Autodesk Fusion 360 part; units mm, degrees
note: some values were not read from the file. Set by a fixed rule: which sketch regions a step uses.
(part 2 of 4)
sketch "Sketch8" plane through (0, 57, 0) normal (0, 1, 0) x (0, 0, 1)
  circle A0 centre (-6, 81) radius 8
  circle A1 centre (-6, 61) radius 8
  circle A2 centre (0, 35) radius 14
  circle A3 centre (0, 0) radius 14
  line L0 (-3, 62.5) -> (-9, 62.5)
  line L1 (-9, 62.5) -> (-9, 59.5)
  line L2 (-9, 59.5) -> (-3, 59.5)
  line L3 (-3, 59.5) -> (-3, 62.5)
  line L4 (-3, 82.5) -> (-9, 82.5)
  line L5 (-3, 79.5) -> (-3, 82.5)
  line L6 (-9, 79.5) -> (-3, 79.5)
  line L7 (-9, 82.5) -> (-9, 79.5)
  arc A4 (3.3646, 47.557) -> (-3.3646, 47.557) centre (0, 35) ccw
  line L8 (-1.1647, 39.3467) -> (-3.3646, 47.557)
  line L9 (1.1647, 39.3467) -> (3.3646, 47.557)
  arc A5 (1.1647, 39.3467) -> (-1.1647, 39.3467) centre (0, 35) ccw
  arc A6 (3.8971, 37.25) -> (2.25, 38.8971) centre (0, 35) ccw
  line L10 (2.25, 38.8971) -> (6.5, 46.2583)
  arc A7 (11.2583, 41.5) -> (6.5, 46.2583) centre (0, 35) ccw
  line L11 (3.8971, 37.25) -> (11.2583, 41.5)
  line L12 (4.3467, 36.1647) -> (12.557, 38.3646)
  arc A8 (12.557, 31.6354) -> (12.557, 38.3646) centre (0, 35) ccw
  line L13 (4.3467, 33.8353) -> (12.557, 31.6354)
  arc A9 (4.3467, 33.8353) -> (4.3467, 36.1647) centre (0, 35) ccw
  arc A10 (-11.2583, 28.5) -> (-6.5, 23.7417) centre (0, 35) ccw
  arc A11 (-3.3646, 22.443) -> (3.3646, 22.443) centre (0, 35) ccw
  arc A12 (6.5, 23.7417) -> (11.2583, 28.5) centre (0, 35) ccw
  line L14 (3.8971, 32.75) -> (11.2583, 28.5)
  arc A13 (2.25, 31.1029) -> (3.8971, 32.75) centre (0, 35) ccw
  line L15 (2.25, 31.1029) -> (6.5, 23.7417)
  arc A14 (-1.1647, 30.6533) -> (1.1647, 30.6533) centre (0, 35) ccw
  line L16 (1.1647, 30.6533) -> (3.3646, 22.443)
  line L17 (-1.1647, 30.6533) -> (-3.3646, 22.443)
  line L18 (-2.25, 31.1029) -> (-6.5, 23.7417)
  line L19 (-3.8971, 32.75) -> (-11.2583, 28.5)
  arc A15 (-3.8971, 32.75) -> (-2.25, 31.1029) centre (0, 35) ccw
  arc A16 (-4.3467, 36.1647) -> (-4.3467, 33.8353) centre (0, 35) ccw
  line L20 (-4.3467, 33.8353) -> (-12.557, 31.6354)
  line L21 (-4.3467, 36.1647) -> (-12.557, 38.3646)
  arc A17 (-12.557, 38.3646) -> (-12.557, 31.6354) centre (0, 35) ccw
  arc A18 (-6.5, 46.2583) -> (-11.2583, 41.5) centre (0, 35) ccw
  line L22 (-2.25, 38.8971) -> (-6.5, 46.2583)
  line L23 (-3.8971, 37.25) -> (-11.2583, 41.5)
  arc A19 (-2.25, 38.8971) -> (-3.8971, 37.25) centre (0, 35) ccw
  line L24 (3, 36.5) -> (-3, 36.5)
  line L25 (-3, 36.5) -> (-3, 33.5)
  line L26 (-3, 33.5) -> (3, 33.5)
  line L27 (3, 33.5) -> (3, 36.5)
  arc A20 (-3.8971, -2.25) -> (-2.25, -3.8971) centre (0, 0) ccw
  arc A21 (-1.1647, -4.3467) -> (1.1647, -4.3467) centre (0, 0) ccw
  arc A22 (2.25, -3.8971) -> (3.8971, -2.25) centre (0, 0) ccw
  arc A23 (4.3467, -1.1647) -> (4.3467, 1.1647) centre (0, 0) ccw
  arc A24 (3.8971, 2.25) -> (2.25, 3.8971) centre (0, 0) ccw
  arc A25 (1.1647, 4.3467) -> (-1.1647, 4.3467) centre (0, 0) ccw
  arc A26 (-2.25, 3.8971) -> (-3.8971, 2.25) centre (0, 0) ccw
  arc A27 (-4.3467, 1.1647) -> (-4.3467, -1.1647) centre (0, 0) ccw
  line L28 (-4.3467, -1.1647) -> (-12.557, -3.3646)
  line L29 (-4.3467, 1.1647) -> (-12.557, 3.3646)
  arc A28 (-12.557, 3.3646) -> (-12.557, -3.3646) centre (0, 0) ccw
  line L30 (-3.8971, -2.25) -> (-11.2583, -6.5)
  arc A29 (-11.2583, -6.5) -> (-6.5, -11.2583) centre (0, 0) ccw
  line L31 (-2.25, -3.8971) -> (-6.5, -11.2583)
  line L32 (-1.1647, -4.3467) -> (-3.3646, -12.557)
  arc A30 (-3.3646, -12.557) -> (3.3646, -12.557) centre (0, 0) ccw
  line L33 (1.1647, -4.3467) -> (3.3646, -12.557)
  line L34 (2.25, -3.8971) -> (6.5, -11.2583)
  arc A31 (6.5, -11.2583) -> (11.2583, -6.5) centre (0, 0) ccw
  line L35 (3.8971, -2.25) -> (11.2583, -6.5)
  line L36 (4.3467, -1.1647) -> (12.557, -3.3646)
  line L37 (4.3467, 1.1647) -> (12.557, 3.3646)
  arc A32 (12.557, -3.3646) -> (12.557, 3.3646) centre (0, 0) ccw
  line L38 (3.8971, 2.25) -> (11.2583, 6.5)
  line L39 (2.25, 3.8971) -> (6.5, 11.2583)
  line L40 (1.1647, 4.3467) -> (3.3646, 12.557)
  line L41 (-1.1647, 4.3467) -> (-3.3646, 12.557)
  line L42 (-2.25, 3.8971) -> (-6.5, 11.2583)
  line L43 (-3.8971, 2.25) -> (-11.2583, 6.5)
  arc A33 (-6.5, 11.2583) -> (-11.2583, 6.5) centre (0, 0) ccw
  arc A34 (3.3646, 12.557) -> (-3.3646, 12.557) centre (0, 0) ccw
  arc A35 (11.2583, 6.5) -> (6.5, 11.2583) centre (0, 0) ccw
  circle A36 centre (0, -35) radius 14
  line L44 (3, -33.5) -> (-3, -33.5)
  line L45 (-3, -33.5) -> (-3, -36.5)
  line L46 (-3, -36.5) -> (3, -36.5)
  line L47 (3, -36.5) -> (3, -33.5)
  arc A37 (4.3467, -36.1647) -> (4.3467, -33.8353) centre (0, -35) ccw
  line L48 (4.3467, -33.8353) -> (12.557, -31.6354)
  arc A38 (12.557, -38.3646) -> (12.557, -31.6354) centre (0, -35) ccw
  line L49 (4.3467, -36.1647) -> (12.557, -38.3646)
  line L50 (3.8971, -37.25) -> (11.2583, -41.5)
  arc A39 (2.25, -38.8971) -> (3.8971, -37.25) centre (0, -35) ccw
  line L51 (2.25, -38.8971) -> (6.5, -46.2583)
  arc A40 (6.5, -46.2583) -> (11.2583, -41.5) centre (0, -35) ccw
  arc A41 (-3.3646, -47.557) -> (3.3646, -47.557) centre (0, -35) ccw
  line L52 (-1.1647, -39.3467) -> (-3.3646, -47.557)
  arc A42 (-1.1647, -39.3467) -> (1.1647, -39.3467) centre (0, -35) ccw
  line L53 (1.1647, -39.3467) -> (3.3646, -47.557)
  line L54 (-2.25, -38.8971) -> (-6.5, -46.2583)
  arc A43 (-11.2583, -41.5) -> (-6.5, -46.2583) centre (0, -35) ccw
  line L55 (-3.8971, -37.25) -> (-11.2583, -41.5)
  arc A44 (-3.8971, -37.25) -> (-2.25, -38.8971) centre (0, -35) ccw
  line L56 (-4.3467, -36.1647) -> (-12.557, -38.3646)
  arc A45 (-12.557, -31.6354) -> (-12.557, -38.3646) centre (0, -35) ccw
  line L57 (-4.3467, -33.8353) -> (-12.557, -31.6354)
  arc A46 (-4.3467, -33.8353) -> (-4.3467, -36.1647) centre (0, -35) ccw
  arc A47 (-2.25, -31.1029) -> (-3.8971, -32.75) centre (0, -35) ccw
  arc A48 (1.1647, -30.6533) -> (-1.1647, -30.6533) centre (0, -35) ccw
  arc A49 (3.8971, -32.75) -> (2.25, -31.1029) centre (0, -35) ccw
  line L58 (-3.8971, -32.75) -> (-11.2583, -28.5)
  arc A50 (-6.5, -23.7417) -> (-11.2583, -28.5) centre (0, -35) ccw
  line L59 (-2.25, -31.1029) -> (-6.5, -23.7417)
  line L60 (-1.1647, -30.6533) -> (-3.3646, -22.443)
  arc A51 (3.3646, -22.443) -> (-3.3646, -22.443) centre (0, -35) ccw
  line L61 (1.1647, -30.6533) -> (3.3646, -22.443)
  line L62 (2.25, -31.1029) -> (6.5, -23.7417)
  arc A52 (11.2583, -28.5) -> (6.5, -23.7417) centre (0, -35) ccw
  line L63 (3.8971, -32.75) -> (11.2583, -28.5)
  circle A53 centre (-6, -81) radius 8
  circle A54 centre (-6, -61) radius 8
  line L64 (-9, -59.5) -> (-9, -62.5)
  line L65 (-3, -59.5) -> (-9, -59.5)
  line L66 (-3, -62.5) -> (-3, -59.5)
  line L67 (-9, -62.5) -> (-3, -62.5)
  line L68 (-3, -79.5) -> (-9, -79.5)
  line L69 (-3, -82.5) -> (-3, -79.5)
  line L70 (-9, -82.5) -> (-3, -82.5)
  line L71 (-9, -79.5) -> (-9, -82.5)
  line L72 (3, 1.5) -> (3, -1.5)
  line L73 (3, -1.5) -> (-3, -1.5)
  line L74 (-3, -1.5) -> (-3, 1.5)
  line L75 (-3, 1.5) -> (3, 1.5)
extrude "Extrude28" add sketch "Sketch8" along normal blind 3 separate body contours A0 makes body 28
extrude "Extrude29" add sketch "Sketch8" along normal blind 3 separate body contours A1 makes body 29
extrude "Extrude30" add sketch "Sketch8" along normal blind 3 separate body contours A2 makes body 30
extrude "Extrude31" add sketch "Sketch8" along normal blind 3 separate body contours A3 makes body 31
extrude "Extrude32" add sketch "Sketch8" along normal blind 3 separate body contours A36 makes body 32
extrude "Extrude33" add sketch "Sketch8" along normal blind 3 separate body contours A54 makes body 33
extrude "Extrude34" add sketch "Sketch8" along normal blind 3 separate body contours A53 makes body 34
ref_plane "WorkPlane8" through (-61, 60, -6) normal (0, 1, 0) x (0, 0, 1)
sketch "Sketch9" plane through (0, 60, 0) normal (0, 1, 0) x (0, 0, 1)
  line L0 (-6, 82.5) -> (-6, 84.5)
  arc A0 (-5, 85.5) -> (-6, 84.5) centre (-5, 84.5) ccw
  line L1 (0, 85.5) -> (-5, 85.5)
  arc A1 (3, 82.5) -> (0, 85.5) centre (0, 82.5) ccw
  line L2 (3, 59.5) -> (3, 82.5)
  arc A2 (0, 56.5) -> (3, 59.5) centre (0, 59.5) ccw
  line L3 (-5, 56.5) -> (0, 56.5)
  line L4 (-6, 59.5) -> (-6, 57.5)
  arc A3 (-6, 57.5) -> (-5, 56.5) centre (-5, 57.5) ccw
  line L5 (-6, 62.5) -> (-6, 79.5)
  line L6 (-3, 79.5) -> (-3, 82.5)
  line L7 (-3, 59.5) -> (-3, 62.5)
  line L8 (-6, -59.5) -> (-6, -57.5)
  arc A4 (-5, -56.5) -> (-6, -57.5) centre (-5, -57.5) ccw
  line L9 (0, -56.5) -> (-5, -56.5)
  line L10 (-3, -62.5) -> (-3, -59.5)
  arc A5 (3, -59.5) -> (0, -56.5) centre (0, -59.5) ccw
  line L11 (3, -82.5) -> (3, -59.5)
  line L12 (-6, -79.5) -> (-6, -62.5)
  line L13 (-3, -82.5) -> (-3, -79.5)
  line L14 (-6, -82.5) -> (-6, -84.5)
  arc A6 (-6, -84.5) -> (-5, -85.5) centre (-5, -84.5) ccw
  line L15 (-5, -85.5) -> (0, -85.5)
  arc A7 (0, -85.5) -> (3, -82.5) centre (0, -82.5) ccw
  line L16 (-3, 82.5) -> (-6, 82.5)
  line L17 (-3, 79.5) -> (-6, 79.5)
  line L18 (-3, 62.5) -> (-6, 62.5)
  line L19 (-3, 59.5) -> (-6, 59.5)
  line L20 (-3, -59.5) -> (-6, -59.5)
  line L21 (-3, -62.5) -> (-6, -62.5)
  line L22 (-3, -79.5) -> (-6, -79.5)
  line L23 (-3, -82.5) -> (-6, -82.5)
  arc A8 (14.7459, 42.5217) -> (16.2941, 44.7585) centre (15, 44) ccw
  line L24 (3.3176, 38.2212) -> (14.7459, 42.5217)
  line L25 (2.2907, 39.2175) -> (15, 44)
  arc A9 (2.2907, 39.2175) -> (-0.2332, 37.8932) centre (1.2462, 38.1409) ccw
  line L26 (0, 36.5) -> (-0.2332, 37.8932)
  line L27 (2.9851, 36.5) -> (0, 36.5)
  line L28 (2.9851, 36.5) -> (2.9851, 33.5)
  line L29 (2.9851, 33.5) -> (0.5022, 33.5)
  arc A10 (0.5208, 33.389) -> (1.0114, 32.179) centre (3.4796, 33.8843) ccw
  line L30 (0.5208, 33.389) -> (0.5022, 33.5)
  line L31 (5.5685, 36.0375) -> (3.3176, 38.2212)
  arc A11 (2.3055, 31.1236) -> (5.5685, 36.0375) centre (3.4796, 33.8843) ccw
  line L32 (2.3055, 4.2031) -> (2.3055, 31.1236)
  line L33 (1.0114, 4.6224) -> (1.0114, 32.179)
  line L34 (2.9851, 1.5) -> (0, 1.5)
  line L35 (0, 1.5) -> (-0.2332, 2.8932)
  arc A12 (1.0114, 4.6224) -> (-0.2332, 2.8932) centre (1.2462, 3.1409) ccw
  line L36 (5.5685, 1.0375) -> (2.2907, 4.2175)
  arc A13 (2.3055, -3.8764) -> (5.5685, 1.0375) centre (3.4796, -1.1157) ccw
  line L37 (2.9851, 1.5) -> (2.9851, -1.5)
  line L38 (2.9851, -1.5) -> (0.5022, -1.5)
  arc A14 (0.5208, -1.611) -> (1.0114, -2.821) centre (3.4796, -1.1157) ccw
  line L39 (0.5208, -1.611) -> (0.5022, -1.5)
  line L40 (1.0114, -30.38) -> (1.0114, -2.821)
  line L41 (2.3055, -30.7825) -> (2.3055, -3.8764)
  line L42 (0.0149, -33.5) -> (-0.2184, -32.1068)
  arc A15 (1.0114, -30.38) -> (-0.2184, -32.1068) centre (1.261, -31.8591) ccw
  line L43 (5.5834, -33.9625) -> (2.3055, -30.7825)
  line L44 (3, -33.5) -> (0.0149, -33.5)
  line L45 (3, -33.5) -> (3, -36.5)
  line L46 (3, -36.5) -> (0.517, -36.5)
  arc A16 (0.5356, -36.611) -> (5.5834, -33.9625) centre (3.4944, -36.1157) ccw
  line L47 (0.5356, -36.611) -> (0.517, -36.5)
  line L48 (15, 78) -> (16.2941, 78)
  line L49 (16.2941, 78) -> (16.2941, 44.7585)
  line L50 (15, 78) -> (15, 44)
  constraint coincident L6.end L16.start
  constraint coincident L0.start L16.end
  constraint coincident L6.start L17.start
  constraint coincident L5.end L17.end
  constraint coincident L7.end L18.start
  constraint coincident L5.start L18.end
  constraint coincident L7.start L19.start
  constraint coincident L4.start L19.end
  constraint coincident L10.end L20.start
  constraint coincident L8.start L20.end
  constraint coincident L10.start L21.start
  constraint coincident L12.end L21.end
  constraint coincident L13.end L22.start
  constraint coincident L12.start L22.end
  constraint coincident L13.start L23.start
  constraint coincident L14.start L23.end
  constraint coincident A8.end L49.end
  constraint perpendicular L48 L49
  constraint coincident A8.centre L25.end
  constraint perpendicular L48 L50
extrude "Extrude35" add sketch "Sketch9" along normal blind 3 separate body contours L8 A4 L9 L10 A5 L11 L12 L13 L14 A6 L15 A7 L20 L21 L22 L23 makes body 35
extrude "Extrude36" add sketch "Sketch9" along normal blind 3 separate body contours L0 A0 L1 A1 L2 A2 L3 L4 A3 L5 L6 L7 L16 L17 L18 L19 makes body 36
extrude "Extrude37" add sketch "Sketch9" along normal blind 3 separate body contours A8 L24 L25 A9 L26 L27 L28 L29 A10 L30 L31 A11 L32 L33 L34 L35 A12 L36 A13 L37 L38 A14 L39 L40 L41 L42 A15 L43 L44 L45 L46 A16 L47 L48 L49 L50 makes body 37
ref_plane "WorkPlane9" through (-59.5, -6, 11.5) normal (0, -1, 0) x (1, 0, 0)
sketch "Sketch10" plane through (0, -6, 0) normal (0, -1, 0) x (1, 0, 0)
  line L0 (-61, 10) -> (-61, 13)
  line L1 (-58, 10) -> (-61, 10)
  line L2 (-58, 10) -> (-58, 13)
  line L3 (-58, 13) -> (-55, 13)
  line L4 (-93, 10) -> (-93, 13)
  line L5 (-93, 10) -> (-90, 10)
  line L6 (-90, 10) -> (-90, 13)
  line L7 (-98, 13) -> (-93, 13)
  line L8 (-90, 13) -> (-61, 13)
  line L9 (-55, 13) -> (-55, 18)
  line L10 (-55, 68) -> (-58, 68)
  line L11 (-58, 68) -> (-58, 65)
  line L12 (-58, 65) -> (-55, 65)
  line L13 (-55, 18) -> (-58, 18)
  line L14 (-58, 18) -> (-58, 21)
  line L15 (-58, 21) -> (-55, 21)
  line L16 (-55, 65) -> (-55, 21)
  line L17 (-98, 13) -> (-98, 18)
  line L18 (-98, 18) -> (-95, 18)
  line L19 (-95, 18) -> (-95, 21)
  line L20 (-95, 21) -> (-98, 21)
  line L21 (-98, 65) -> (-98, 21)
  line L22 (-95, 65) -> (-98, 65)
  line L23 (-95, 68) -> (-95, 65)
  line L24 (-98, 68) -> (-95, 68)
  line L25 (-88.5, 67.3205) -> (-64.5, 67.3205)
  arc A0 (-88.5, 67.3205) -> (-91.5, 64.3205) centre (-88.5, 64.3205) ccw
  arc A1 (-61.5, 64.3205) -> (-64.5, 67.3205) centre (-64.5, 64.3205) ccw
  line L26 (-91.5, 64.3205) -> (-91.5, 47.3205)
  line L27 (-61.5, 64.3205) -> (-61.5, 47.3205)
  line L28 (-64.5, 44.3205) -> (-88.5, 44.3205)
  arc A2 (-91.5, 47.3205) -> (-88.5, 44.3205) centre (-88.5, 47.3205) ccw
  arc A3 (-64.5, 44.3205) -> (-61.5, 47.3205) centre (-64.5, 47.3205) ccw
  line L29 (-98, 68) -> (-98, 70)
  line L30 (-55, 68) -> (-55, 70)
  line L31 (-55, 70) -> (-98, 70)
  point P0 (-93, 68)
  point P1 (-60, 68)
  point P2 (-60, 29)
  point P3 (-93, 29)
  point P4 (-91.5, 67.3205)
  point P5 (-61.5, 67.3205)
  point P6 (-91.5, 44.3205)
  point P7 (-61.5, 44.3205)
  dimension "d185" = 39
  dimension "d186" = 39
  dimension "d191" = 5
  dimension "d193" = 3
  dimension "d194" = 3
  dimension "d195" = 3
  dimension "d197" = 3
  dimension "d198" = 3
  dimension "d199" = 30
  dimension "d202" = 3
  dimension "d203" = 3
  dimension "d208" = 20
  dimension "d209" = 20
  dimension "d210" = 3
  dimension "d211" = 3
  dimension "d271" = 2
  dimension "d272" = 2
  constraint coincident L3.end L9.start
  constraint perpendicular L3 L9
  constraint perpendicular L10 L11
  constraint perpendicular L11 L12
  constraint horizontal L13
  constraint perpendicular L13 L14
  constraint perpendicular L14 L15
  constraint horizontal L25
  constraint coincident P4 L25
  constraint tangent L25 A0
  constraint coincident P5 L25
  constraint tangent L25 A1
  constraint vertical L26
  constraint vertical L27
  constraint perpendicular L26 L28
  constraint coincident P6 L26
  constraint coincident P6 L28
  constraint tangent L26 A2
  constraint tangent L28 A2
  constraint coincident P7 L28
  constraint coincident P7 L27
  constraint tangent L28 A3
  constraint tangent L27 A3
  constraint perpendicular L24 L29
  measures "d185" distance of P1 P2
  measures "d186" distance of P0 P3
  measures "d191" distance of L3.end L9.end
  measures "d193" distance of L10.start L10.end
  measures "d194" distance of L10.end L11.end
  measures "d195" distance of L11.end L12.end
  measures "d197" distance of L9.end L13.end
  measures "d198" distance of L14.end L15.end
  measures "d199" distance of P4 P5
  measures "d202" radius of A0
  measures "d203" radius of A1
  measures "d208" distance of A0.end P6
  measures "d209" distance of A1.start P7
  measures "d210" radius of A2
  measures "d211" radius of A3
  measures "d271" distance of L24.start L29.end
  measures "d272" distance of L10.start L30.end
extrude "Extrude38" add sketch "Sketch10" along normal blind 3 separate body makes body 38
ref_plane "WorkPlane10" through (-61.5, 60, 11.5) normal (0, 1, 0) x (-1, 0, 0)
sketch "Sketch11" plane through (0, 60, 0) normal (0, 1, 0) x (-1, 0, 0)
  arc A0 (91.5, 64.3205) -> (88.5, 67.3205) centre (88.5, 64.3205) ccw
  line L0 (91.5, 64.3205) -> (91.5, 47.3205)
  arc A1 (88.5, 44.3205) -> (91.5, 47.3205) centre (88.5, 47.3205) ccw
  line L1 (88.5, 44.3205) -> (64.5, 44.3205)
  arc A2 (61.5, 47.3205) -> (64.5, 44.3205) centre (64.5, 47.3205) ccw
  line L2 (61.5, 47.3205) -> (61.5, 64.3205)
  arc A3 (64.5, 67.3205) -> (61.5, 64.3205) centre (64.5, 64.3205) ccw
  line L3 (64.5, 67.3205) -> (88.5, 67.3205)
  line L4 (55, 68) -> (58, 68)
  line L5 (58, 68) -> (58, 65)
  line L6 (58, 65) -> (55, 65)
  line L7 (55, 65) -> (55, 21)
  line L8 (55, 21) -> (58, 21)
  line L9 (58, 21) -> (58, 18)
  line L10 (58, 18) -> (55, 18)
  line L11 (55, 18) -> (55, 13)
  line L12 (55, 13) -> (58, 13)
  line L13 (58, 13) -> (58, 10)
  line L14 (58, 10) -> (61, 10)
  line L15 (61, 10) -> (61, 13)
  line L16 (61, 13) -> (90, 13)
  line L17 (90, 13) -> (90, 10)
  line L18 (90, 10) -> (93, 10)
  line L19 (93, 10) -> (93, 13)
  line L20 (93, 13) -> (98, 13)
  line L21 (98, 13) -> (98, 18)
  line L22 (98, 18) -> (95, 18)
  line L23 (95, 18) -> (95, 21)
  line L24 (95, 21) -> (98, 21)
  line L25 (98, 21) -> (98, 65)
  line L26 (98, 65) -> (95, 65)
  line L27 (95, 65) -> (95, 68)
  line L28 (95, 68) -> (98, 68)
  line L29 (55, 68) -> (55, 70)
  line L30 (98, 68) -> (98, 70)
  line L31 (98, 70) -> (55, 70)
  line L32 (55, 70) -> (55, 68)
  line L33 (98, 68) -> (98, 70)
  line L34 (98, 70) -> (55, 70)
  dimension "d269" = 2
  dimension "d270" = 2
  constraint coincident L4.start L29.start
  constraint perpendicular L6 L29
  constraint coincident L28.end L30.start
  constraint perpendicular L28 L30
  measures "d269" distance of L4.start L29.end
  measures "d270" distance of L28.end L30.end
extrude "Extrude39" add sketch "Sketch11" along normal blind 3 separate body makes body 39
ref_plane "WorkPlane11" through (-95, -7.5, 66.5) normal (-1, 0, 0) x (0, 0, -1)
sketch "Sketch12" plane through (-95, 0, 0) normal (-1, 0, 0) x (0, 0, -1)
  line L0 (-18, -63) -> (-21, -63)
  line L1 (-21, -60) -> (-21, -63)
  line L2 (-18, -60) -> (-18, -63)
  line L3 (-13, -60) -> (-18, -60)
  line L4 (-10, -58) -> (-13, -58)
  line L5 (-10, -58) -> (-10, -55)
  line L6 (-10, -55) -> (-13, -55)
  line L7 (-13, -55) -> (-13, -28.5)
  line L8 (-13, -25.5) -> (-13, 1)
  line L9 (-10, 1) -> (-13, 1)
  line L10 (-10, 4) -> (-10, 1)
  line L11 (-10, 4) -> (-13, 4)
  line L12 (-13, 6) -> (-18, 6)
  line L13 (-18, 6) -> (-18, 9)
  line L14 (-21, 9) -> (-18, 9)
  line L15 (-21, 6) -> (-21, 9)
  line L16 (-65, 6) -> (-65, 9)
  line L17 (-68, 9) -> (-65, 9)
  line L18 (-68, 6) -> (-68, 9)
  line L19 (-73, 6) -> (-68, 6)
  line L20 (-65, -60) -> (-65, -63)
  line L21 (-65, -63) -> (-68, -63)
  line L22 (-68, -60) -> (-68, -63)
  line L23 (-13, -28.5) -> (-7, -28.5)
  line L24 (-7, -28.5) -> (-7, -25.5)
  line L25 (-13, -25.5) -> (-7, -25.5)
  line L26 (-13, -55) -> (-13, -28.5)
  line L27 (-13, 1) -> (-13, -25.5)
  line L28 (-79.7175, -57.5251) -> (-77.5962, -59.6464)
  line L29 (-77.5962, -59.6464) -> (-75.4749, -57.5251)
  line L30 (-79.7175, -57.5251) -> (-77.5962, -55.4038)
  line L31 (-73, -60) -> (-75.4749, -57.5251)
  line L32 (-77.5962, -55.4038) -> (-80.0711, -52.9289)
  line L33 (-84.1542, -47.0486) -> (-83.6333, -50.003)
  line L34 (-84.1542, -47.0486) -> (-81.1998, -46.5277)
  line L35 (-83.6333, -50.003) -> (-80.6788, -49.4821)
  line L36 (-80.0711, -52.9289) -> (-80.6788, -49.4821)
  line L37 (-81.1998, -46.5277) -> (-81.8075, -43.0809)
  line L38 (-77.5962, 5.6464) -> (-75.4749, 3.5251)
  line L39 (-79.7175, 3.5251) -> (-77.5962, 5.6464)
  line L40 (-79.7175, 3.5251) -> (-77.5962, 1.4038)
  line L41 (-83.6333, -3.9969) -> (-80.6788, -4.5179)
  line L42 (-84.1542, -6.9514) -> (-83.6333, -3.9969)
  line L43 (-84.1542, -6.9514) -> (-81.1998, -7.4723)
  line L44 (-84.8075, -28.5) -> (-84.8075, -25.5)
  line L45 (-84.8075, -25.5) -> (-81.8075, -25.5)
  line L46 (-84.8075, -28.5) -> (-81.8075, -28.5)
  line L47 (-81.8075, -43.0809) -> (-81.8075, -28.5)
  line L48 (-81.8075, -25.5) -> (-81.8075, -10.9191)
  line L49 (-80.0711, -1.0711) -> (-80.6788, -4.5179)
  line L50 (-81.1998, -7.4723) -> (-81.8075, -10.9191)
  line L51 (-73, 6) -> (-75.4749, 3.5251)
  line L52 (-77.5962, 1.4038) -> (-80.0711, -1.0711)
  line L53 (-21, -60) -> (-65, -60)
  line L54 (-65, 6) -> (-21, 6)
  line L55 (-73, 6) -> (-68, 6)
  line L56 (-68, -60) -> (-73, -60)
  line L57 (-13, -60) -> (-13, -58)
  line L58 (-13, 4) -> (-13, 6)
  dimension "d222" = 3
  dimension "d224" = 10
  dimension "d226" = 10
  dimension "d228" = 10
  dimension "d230" = 10
  dimension "d233" = 3
  dimension "d236" = 3
  dimension "d240" = 3
  constraint coincident L7.end L23.start
  constraint perpendicular L7 L23
  constraint perpendicular L23 L24
  constraint coincident L8.start L25.start
  constraint coincident L6.end L7.start
  constraint coincident L8.end L9.end
  constraint coincident L19.start L51.start
  constraint perpendicular L29 L31
  constraint coincident L30.end L31
  constraint perpendicular L30 L31
  constraint collinear L31 L32
  constraint coincident L34.end L36
  constraint perpendicular L34 L36
  constraint perpendicular L35 L36
  constraint collinear L36 L37
  constraint vertical L44
  constraint coincident L45.end L47
  constraint perpendicular L45 L47
  constraint perpendicular L46 L47
  constraint collinear L47 L48
  constraint collinear L49 L50
  constraint collinear L51 L52
  constraint coincident L1.start L53.start
  constraint coincident L20.start L53.end
  constraint coincident L16.start L54.start
  constraint coincident L15.start L54.end
  constraint coincident L18.start L19.end
  constraint coincident L22.start L56.start
  constraint perpendicular L22 L56
  constraint coincident L3.start L57.start
  constraint coincident L4.end L57.end
  constraint coincident L11.end L58.start
  constraint coincident L12.start L58.end
  measures "d222" distance of L23.end L24.end
  measures "d224" distance of L31.start L32.end
  measures "d226" distance of L19.start L49.start
  measures "d228" distance of L32.end L37.end
  measures "d230" distance of L49.start L48.end
  measures "d233" distance of L28.start L28.end
  measures "d236" distance of L33.start L33.end
  measures "d240" distance of L44.start L44.end
extrude "Extrude40" add sketch "Sketch12" along normal blind 3 separate body makes body 40
ref_plane "WorkPlane12" through (-58, -7.5, 66.5) normal (1, 0, 0) x (0, 0, 1)
sketch "Sketch13" plane through (-58, 0, 0) normal (1, 0, 0) x (0, 0, 1)
  line L0 (13, -60) -> (18, -60)
  line L1 (18, -60) -> (18, -63)
  line L2 (18, -63) -> (21, -63)
  line L3 (21, -63) -> (21, -60)
  line L4 (21, -60) -> (65, -60)
  line L5 (65, -60) -> (65, -63)
  line L6 (65, -63) -> (68, -63)
  line L7 (68, -63) -> (68, -60)
  line L8 (68, -60) -> (73, -60)
  line L9 (73, -60) -> (75.4749, -57.5251)
  line L10 (75.4749, -57.5251) -> (77.5962, -59.6464)
  line L11 (77.5962, -59.6464) -> (79.7175, -57.5251)
  line L12 (79.7175, -57.5251) -> (77.5962, -55.4038)
  line L13 (77.5962, -55.4038) -> (80.0711, -52.9289)
  line L14 (80.0711, -52.9289) -> (80.6788, -49.4821)
  line L15 (80.6788, -49.4821) -> (83.6333, -50.003)
  line L16 (83.6333, -50.003) -> (84.1542, -47.0486)
  line L17 (84.1542, -47.0486) -> (81.1998, -46.5277)
  line L18 (81.1998, -46.5277) -> (81.8075, -43.0809)
  line L19 (81.8075, -43.0809) -> (81.8075, -28.5)
  line L20 (81.8075, -28.5) -> (84.8075, -28.5)
  line L21 (84.8075, -28.5) -> (84.8075, -25.5)
  line L22 (84.8075, -25.5) -> (81.8075, -25.5)
  line L23 (81.8075, -25.5) -> (81.8075, -10.9191)
  line L24 (81.8075, -10.9191) -> (81.1998, -7.4723)
  line L25 (81.1998, -7.4723) -> (84.1542, -6.9514)
  line L26 (84.1542, -6.9514) -> (83.6333, -3.9969)
  line L27 (83.6333, -3.9969) -> (80.6788, -4.5179)
  line L28 (80.6788, -4.5179) -> (80.0711, -1.0711)
  line L29 (80.0711, -1.0711) -> (77.5962, 1.4038)
  line L30 (77.5962, 1.4038) -> (79.7175, 3.5251)
  line L31 (79.7175, 3.5251) -> (77.5962, 5.6464)
  line L32 (77.5962, 5.6464) -> (75.4749, 3.5251)
  line L33 (75.4749, 3.5251) -> (73, 6)
  line L34 (73, 6) -> (68, 6)
  line L35 (68, 6) -> (68, 9)
  line L36 (68, 9) -> (65, 9)
  line L37 (65, 9) -> (65, 6)
  line L38 (65, 6) -> (21, 6)
  line L39 (21, 6) -> (21, 9)
  line L40 (21, 9) -> (18, 9)
  line L41 (18, 9) -> (18, 6)
  line L42 (18, 6) -> (13, 6)
  line L43 (13, 6) -> (13, -8)
  line L44 (13, -60) -> (13, -46)
  line L45 (13, -8) -> (10, -8)
  line L46 (10, -8) -> (10, -11)
  line L47 (10, -11) -> (13, -11)
  line L48 (13, -46) -> (10, -46)
  line L49 (10, -46) -> (10, -43)
  line L50 (10, -43) -> (13, -43)
  line L51 (13, -43) -> (13, -11)
  line L52 (76.8075, -9) -> (76.8075, -45)
  line L53 (13, 9) -> (13, 0)
  line L54 (70.8075, -3) -> (49.4645, -3)
  line L55 (70.8075, -51) -> (49.4645, -51)
  arc A0 (76.8075, -9) -> (70.8075, -3) centre (70.8075, -9) ccw
  arc A1 (70.8075, -51) -> (76.8075, -45) centre (70.8075, -45) ccw
  spline S0 degree 5 poles (49.4645, -3) (50.2739, -3.96) (51.822, -5.88) (53.9322, -8.76) (56.3146, -12.6) (58.5253, -17.4) (59.9, -22.2) (60.3707, -27) (59.9, -31.8) (58.5253, -36.6) (56.3146, -41.4) (53.9322, -45.24) (51.822, -48.12) (50.2739, -50.04) (49.4645, -51) knots 0 0 0 0 0 0 0.1 0.2 0.3 0.4 0.5 0.6 0.7 0.8 0.9 1 1 1 1 1 1
  line L56 (18, -6) -> (18, -3)
  line L57 (18, -3) -> (21, -3)
  line L58 (21, -3) -> (21, -6)
  line L59 (21, -6) -> (18, -6)
  line L60 (18, -48) -> (21, -48)
  line L61 (21, -48) -> (21, -51)
  line L62 (21, -51) -> (18, -51)
  line L63 (18, -51) -> (18, -48)
  line L64 (36.4645, -3) -> (36.4645, -6)
  line L65 (36.4645, -6) -> (39.4645, -6)
  line L66 (39.4645, -6) -> (39.4645, -3)
  line L67 (39.4645, -3) -> (36.4645, -3)
  line L68 (39.4645, -51) -> (36.4645, -51)
  line L69 (39.4645, -48) -> (39.4645, -51)
  line L70 (36.4645, -48) -> (39.4645, -48)
  line L71 (36.4645, -51) -> (36.4645, -48)
  line L72 (44.4645, -6) -> (54.4645, -6) construction
  line L73 (44.4645, -48) -> (54.4645, -48) construction
  line L74 (51.5355, -40.9289) -> (59.5355, -40.9289) construction
  line L75 (51.182, -8.4749) -> (49.0607, -10.5962)
  line L76 (49.0607, -10.5962) -> (46.9393, -8.4749)
  line L77 (46.9393, -8.4749) -> (49.0607, -6.3536)
  line L78 (49.0607, -6.3536) -> (51.182, -8.4749)
  line L79 (55.445, -17.9666) -> (52.4906, -18.4875)
  line L80 (52.4906, -18.4875) -> (51.9697, -15.5331)
  line L81 (51.9697, -15.5331) -> (54.9241, -15.0121)
  line L82 (55.445, -17.9666) -> (54.9241, -15.0121)
  line L83 (55.9247, -25.5) -> (55.9247, -28.5)
  line L84 (52.9247, -25.5) -> (52.9247, -28.5)
  line L85 (52.9247, -28.5) -> (55.9247, -28.5)
  line L86 (55.9247, -25.5) -> (52.9247, -25.5)
  line L87 (49.0607, -47.6464) -> (51.182, -45.5251)
  line L88 (51.182, -45.5251) -> (49.0607, -43.4038)
  line L89 (46.9393, -45.5251) -> (49.0607, -47.6464)
  line L90 (49.0607, -43.4038) -> (46.9393, -45.5251)
  line L91 (51.9697, -38.4669) -> (54.9241, -38.9879)
  line L92 (52.4906, -35.5125) -> (51.9697, -38.4669)
  line L93 (55.445, -36.0334) -> (52.4906, -35.5125)
  line L94 (55.445, -36.0334) -> (54.9241, -38.9879)
  point P0 (76.8075, -52.9523)
  point P1 (60.136, -27)
  point P2 (13, -48)
  dimension "d251" = 14
  dimension "d311" = 6
  dimension "d312" = 6
  dimension "d328" = 3
  dimension "d340" = 5
  dimension "d352" = 3
  dimension "d353" = 3
  dimension "d356" = 3
  dimension "d358" = 3
  dimension "d359" = 3
  dimension "d362" = 3
  constraint coincident L42.end L43.start
  constraint perpendicular L42 L43
  constraint coincident L0.start L44.start
  constraint perpendicular L0 L44
  constraint perpendicular L43 L45
  constraint perpendicular L45 L46
  constraint perpendicular L46 L47
  constraint perpendicular L44 L48
  constraint perpendicular L48 L49
  constraint perpendicular L49 L50
  constraint vertical L52
  constraint horizontal L54
  constraint perpendicular L52 L55
  constraint tangent L52 A0
  constraint tangent L54 A0
  constraint tangent L55 A1
  constraint tangent L52 A1
  constraint perpendicular L56 L57
  constraint perpendicular L57 L58
  constraint perpendicular L56 L59
  constraint perpendicular L44 L60
  constraint perpendicular L60 L61
  constraint perpendicular L61 L62
  constraint perpendicular L64 L65
  constraint perpendicular L65 L66
  constraint perpendicular L64 L67
  constraint horizontal L72
  constraint horizontal L73
  constraint horizontal L74
  constraint perpendicular L75 L76
  constraint perpendicular L76 L77
  constraint perpendicular L75 L78
  constraint perpendicular L79 L80
  constraint perpendicular L80 L81
  constraint vertical L83
  constraint perpendicular L83 L85
  measures "d251" distance of L0.start L44.end
  measures "d311" radius of A0
  measures "d312" radius of A1
  measures "d328" distance of L64.end L65.end
  measures "d340" distance of L65.end L72.start
  measures "d352" distance of L75.end L76.end
  measures "d353" distance of L76.end L77.end
  measures "d356" distance of L79.start L79.end
  measures "d358" distance of L79.end L80.end
  measures "d359" distance of L80.end L81.end
  measures "d361" distance of L83.start L83.end
  measures "d362" distance of L83
extrude "Extrude41" add sketch "Sketch13" along normal blind 3 separate body makes body 41
ref_plane "WorkPlane13" through (-96.5, 54.1664, 78.8336) normal (0, 0.707107, 0.707107) x (0, 0.707107, -0.707107)
sketch "Sketch14" plane through (0, 66.5, 66.5) normal (0, 0.707107, 0.707107) x (0, 0.707107, -0.707107)
  line L0 (-19.1924, 103) -> (-19.1924, 50)
  line L1 (-12.6924, 98) -> (-15.6924, 98)
  line L2 (-15.6924, 98) -> (-15.6924, 95)
  line L3 (-15.6924, 95) -> (-12.6924, 95)
  line L4 (-12.6924, 95) -> (-12.6924, 98)
  line L5 (-12.6924, 55) -> (-15.6924, 55)
  line L6 (-15.6924, 55) -> (-15.6924, 58)
  line L7 (-12.6924, 55) -> (-12.6924, 58)
  line L8 (-12.6924, 58) -> (-15.6924, 58)
  line L9 (-4.1924, 103) -> (-4.1924, 50)
  line L10 (-19.1924, 103) -> (-4.1924, 103)
  line L11 (-4.1924, 50) -> (-19.1924, 50)
  point P0 (-12.6924, 55)
  point P1 (-15.6924, 55)
  point P2 (-15.6924, 98)
  point P3 (-12.6924, 98)
  dimension "d263" = 3
  constraint coincident P3 L1.start
  constraint coincident P2 L1.end
  constraint perpendicular L1 L2
  constraint perpendicular L2 L3
  constraint perpendicular L1 L4
  constraint coincident P0 L5.start
  constraint coincident P1 L5.end
  constraint perpendicular L5 L6
  constraint perpendicular L5 L7
  constraint perpendicular L9 L10
  constraint perpendicular L0 L11
  measures "d263" distance of P1 L6.end
extrude "Extrude42" add sketch "Sketch14" along normal blind 3 separate body makes body 42
ref_plane "WorkPlane14" through (-96.5, -0.1664, 78.8336) normal (0, -0.707107, 0.707107) x (0, 0.707107, 0.707107)
sketch "Sketch15" plane through (0, -39.5, 39.5) normal (0, -0.707107, 0.707107) x (0, 0.707107, 0.707107)
  line L0 (53.8762, 55) -> (50.8762, 55)
  line L1 (50.8762, 55) -> (50.8762, 58)
  line L2 (50.8762, 58) -> (53.8762, 58)
  line L3 (53.8762, 58) -> (53.8762, 55)
  line L4 (57.3762, 55) -> (57.3762, 50)
  line L5 (57.3762, 50) -> (43.3762, 50)
  line L6 (57.3762, 103) -> (43.3762, 103)
  line L7 (43.3762, 50) -> (43.3762, 103)
  line L8 (57.3762, 55) -> (57.3762, 103)
  line L9 (53.8762, 98) -> (53.8762, 95)
  line L10 (53.8762, 95) -> (53.8762, 98)
  line L11 (53.8762, 98) -> (50.8762, 98)
  line L12 (53.8762, 95) -> (50.8762, 95)
  line L13 (50.8762, 98) -> (50.8762, 95)
  point P0 (53.8762, 98)
  point P1 (50.8762, 55)
  point P2 (53.8762, 55)
  point P3 (57.3762, 55)
  dimension "d274" = 5
  dimension "d275" = 14
  dimension "d277" = 14
  dimension "d278" = 3
  constraint coincident P2 L0.start
  constraint coincident P1 L0.end
  constraint perpendicular L0 L1
  constraint perpendicular L1 L2
  constraint perpendicular L0 L3
  constraint coincident P3 L4.start
  constraint perpendicular L0 L4
  constraint perpendicular L4 L5
  constraint perpendicular L6 L8
  constraint coincident P0 L9.start
  constraint perpendicular L6 L9
  constraint perpendicular L6 L10
  constraint perpendicular L10 L11
  constraint perpendicular L10 L12
  constraint perpendicular L11 L13
  measures "d274" distance of P3 L4.end
  measures "d275" distance of L4.end L5.end
  measures "d277" distance of L6.start L6.end
  measures "d278" distance of P0 L11.end
extrude "Extrude43" add sketch "Sketch15" along normal blind 3 separate body makes body 43
ref_plane "WorkPlane15" through (-96.5, 44.8043, 81.5037) normal (0, 0.173648, 0.984808) x (0, 0.984808, -0.173648)
sketch "Sketch16" plane through (0, 15.289, 86.708) normal (0, 0.173648, 0.984808) x (0, 0.984808, -0.173648)
  line L0 (34.7206, 55) -> (31.7206, 55)
  line L1 (34.7206, 55) -> (34.7206, 58)
  line L2 (34.7206, 58) -> (31.7206, 58)
  line L3 (31.7206, 55) -> (31.7206, 58)
  line L4 (34.7206, 98) -> (31.7206, 98)
  line L5 (31.7206, 98) -> (31.7206, 95)
  line L6 (31.7206, 95) -> (34.7206, 95)
  line L7 (34.7206, 95) -> (34.7206, 98)
  line L8 (28.2206, 103) -> (38.2206, 103)
  line L9 (28.2206, 50) -> (38.2206, 50)
  line L10 (38.2206, 50) -> (38.2206, 103)
  line L11 (28.2206, 50) -> (28.2206, 103)
  point P0 (34.7206, 98)
  point P1 (34.7206, 95)
  point P2 (31.7206, 95)
  point P3 (31.7206, 98)
  point P4 (34.7206, 58)
  point P5 (34.7206, 55)
  point P6 (31.7206, 55)
  point P7 (31.7206, 58)
  dimension "d283" = 10
  dimension "d284" = 10
  constraint coincident P5 L0.start
  constraint coincident P6 L0.end
  constraint coincident P4 L1.end
  constraint coincident P7 L2.end
  constraint coincident P0 L4.start
  constraint coincident P3 L4.end
  constraint coincident P2 L5.end
  constraint coincident P1 L6.end
  constraint horizontal L8
  constraint perpendicular L8 L10
  constraint perpendicular L8 L11
  measures "d283" distance of L8.start L8.end
  measures "d284" distance of L9.start L9.end
extrude "Extrude44" add sketch "Sketch16" along normal blind 3 separate body makes body 44
ref_plane "WorkPlane16" through (-96.5, 2.7945, 80.375) normal (0, -0.173648, 0.984808) x (0, 0.984808, 0.173648)
sketch "Sketch17" plane through (0, -13.6607, 77.4735) normal (0, -0.173648, 0.984808) x (0, 0.984808, 0.173648)
  line L0 (18.459, 95) -> (18.459, 98)
  line L1 (18.459, 98) -> (21.459, 98)
  line L2 (21.459, 95) -> (18.459, 95)
  line L3 (21.459, 55) -> (21.459, 58)
  line L4 (21.459, 58) -> (18.459, 58)
  line L5 (18.459, 58) -> (18.459, 55)
  line L6 (18.459, 55) -> (21.459, 55)
  line L7 (24.959, 50) -> (14.959, 50)
  line L8 (24.959, 103) -> (14.959, 103)
  line L9 (14.959, 103) -> (14.959, 50)
  line L10 (24.959, 103) -> (24.959, 50)
  point P0 (18.459, 98)
  point P1 (21.459, 98)
  point P2 (21.459, 95)
  point P3 (18.459, 95)
  point P4 (21.459, 55)
  point P5 (18.459, 55)
  point P6 (18.459, 58)
  point P7 (21.459, 58)
  dimension "d288" = 10
  dimension "d290" = 10
  constraint coincident P3 L0.start
  constraint coincident P0 L0.end
  constraint coincident P1 L1.end
  constraint coincident P2 L2.start
  constraint coincident P4 L3.start
  constraint coincident P7 L3.end
  constraint coincident P6 L4.end
  constraint coincident P5 L5.end
  constraint perpendicular L7 L9
  constraint perpendicular L7 L10
  measures "d288" distance of L7.start L7.end
  measures "d290" distance of L8.start L8.end
extrude "Extrude45" add sketch "Sketch17" along normal blind 3 separate body makes body 45
ref_plane "WorkPlane17" through (-56.5, 18.2096, 81.8075) normal (0, 0, 1) x (0, -1, 0)
sketch "Sketch18" plane through (0, 0, 81.8075) normal (0, 0, 1) x (0, -1, 0)
  line L0 (-28.5, -98) -> (-25.5, -98)
  line L1 (-25.5, -98) -> (-25.5, -95)
  line L2 (-25.5, -95) -> (-25.5, -98)
  line L3 (-25.5, -95) -> (-28.5, -95)
  line L4 (-28.5, -95) -> (-28.5, -98)
  line L5 (-28.5, -58) -> (-25.5, -58)
  line L6 (-25.5, -58) -> (-25.5, -55)
  line L7 (-25.5, -55) -> (-28.5, -55)
  line L8 (-28.5, -55) -> (-28.5, -58)
  line L9 (-10.9191, -50) -> (-43.0809, -50)
  line L10 (-43.0809, -103) -> (-10.9191, -103)
  line L11 (-43.0809, -50) -> (-43.0809, -103)
  line L12 (-10.9191, -50) -> (-10.9191, -103)
  point P0 (-28.5, -98)
  point P1 (-28.5, -95)
  point P2 (-25.5, -95)
  point P3 (-25.5, -98)
  point P4 (-28.5, -58)
  point P5 (-28.5, -55)
  point P6 (-25.5, -55)
  point P7 (-25.5, -58)
  constraint coincident P0 L0.start
  constraint coincident P3 L0.end
  constraint coincident P2 L1.end
  constraint coincident P1 L3.end
  constraint coincident P4 L5.start
  constraint coincident P7 L5.end
  constraint coincident P6 L6.end
  constraint coincident P5 L7.end
  constraint perpendicular L10 L11
  constraint perpendicular L10 L12
extrude "Extrude46" add sketch "Sketch18" along normal blind 3 separate body makes body 46
ref_plane "WorkPlane18" through (-6, 6, 11.5) normal (0, -1, 0) x (1, 0, 0)
sketch "Sketch19" plane through (0, 6, 0) normal (0, -1, 0) x (-1, 0, 0)
  line L0 (36.5, -10) -> (36.5, -13)
  line L1 (33.5, -10) -> (33.5, -13)
  line L2 (36.5, -10) -> (33.5, -10)
  line L3 (4.5, -10) -> (4.5, -13)
  line L4 (7.5, -10) -> (4.5, -10)
  line L5 (7.5, -10) -> (7.5, -13)
  line L6 (-21.5, -10) -> (-21.5, -13)
  line L7 (-21.5, -10) -> (-24.5, -10)
  line L8 (-24.5, -10) -> (-24.5, -13)
  line L9 (-50.5, -10) -> (-53.5, -10)
  line L10 (-53.5, -10) -> (-53.5, -13)
  line L11 (-50.5, -10) -> (-50.5, -13)
  line L12 (58, -18) -> (55, -18)
  line L13 (58, -36.4645) -> (55, -36.4645)
  line L14 (55, -18) -> (55, -13)
  line L15 (55, -13) -> (36.5, -13)
  line L16 (33.5, -13) -> (7.5, -13)
  line L17 (4.5, -13) -> (-21.5, -13)
  line L18 (-24.5, -13) -> (-50.5, -13)
  line L19 (-53.5, -13) -> (-84, -13)
  line L20 (58, -18) -> (58, -21)
  line L21 (58, -21) -> (55, -21)
  line L22 (55, -21) -> (55, -36.4645)
  line L23 (58, -36.4645) -> (58, -39.4645)
  line L24 (58, -39.4645) -> (55, -39.4645)
  line L25 (55, -39.4645) -> (55, -44.4645)
  line L26 (55, -44.4645) -> (-84, -44.4645)
  line L27 (-81, -30.2322) -> (-81, -27.2322)
  line L28 (-81, -30.2322) -> (-84, -30.2322)
  line L29 (-81, -27.2322) -> (-84, -27.2322)
  line L30 (-84, -44.4645) -> (-84, -30.2322)
  line L31 (-84, -27.2322) -> (-84, -13)
  line L32 (-78, -16.2941) -> (-78, -15)
  line L33 (-78, -15) -> (-60, -15)
  line L34 (-78, -16.2941) -> (-60, -16.2941)
  line L35 (-60, -15) -> (-60, -16.2941)
  point P0 (55, -13)
  point P1 (-68, -13)
  point P2 (-80.2343, -13)
  dimension "d330" = 3
  dimension "d331" = 3
  dimension "d332" = 3
  dimension "d333" = 3
  dimension "d334" = 5
  dimension "d363" = 139
  dimension "d614" = 18
  dimension "d615" = 18
  constraint coincident L12.end L14.start
  constraint coincident P0 L14.end
  constraint coincident L0.end L15.end
  constraint coincident L1.end L16.start
  constraint coincident L5.end L16.end
  constraint coincident L3.end L17.start
  constraint coincident L6.end L17.end
  constraint coincident L8.end L18.start
  constraint coincident L11.end L18.end
  constraint coincident L10.end L19.start
  constraint coincident L12.start L20.start
  constraint perpendicular L12 L20
  constraint perpendicular L20 L21
  constraint coincident L13.end L22.end
  constraint coincident L13.start L23.start
  constraint perpendicular L13 L23
  constraint perpendicular L23 L24
  constraint perpendicular L24 L25
  constraint perpendicular L25 L26
  constraint perpendicular L19 L30
  constraint vertical L27
  constraint perpendicular L28 L30
  constraint coincident L29.end L30
  constraint perpendicular L29 L30
  constraint collinear L30 L31
  constraint perpendicular L32 L33
  constraint horizontal L34
  measures "d330" distance of L12.start L20.end
  measures "d331" distance of L20.end L21.end
  measures "d332" distance of L13.start L23.end
  measures "d333" distance of L23.end L24.end
  measures "d334" distance of L24.end L25.end
  measures "d363" distance of L25.end L26.end
  measures "d614" distance of L32.end L33.end
  measures "d615" distance of L32.start L34.end
extrude "Extrude47" add sketch "Sketch19" along normal blind 3 separate body makes body 47
ref_plane "WorkPlane19" through (23, 48, 11.5) normal (0, 1, 0) x (-1, 0, 0)
sketch "Sketch20" plane through (0, 48, 0) normal (0, 1, 0) x (-1, 0, 0)
  line L0 (55, 36.4645) -> (58, 36.4645)
  line L1 (58, 36.4645) -> (58, 39.4645)
  line L2 (58, 39.4645) -> (55, 39.4645)
  line L3 (55, 39.4645) -> (55, 44.4645)
  line L4 (55, 44.4645) -> (-84, 44.4645)
  line L5 (-84, 13) -> (-53.5, 13)
  line L6 (-53.5, 13) -> (-53.5, 10)
  line L7 (-53.5, 10) -> (-50.5, 10)
  line L8 (-50.5, 10) -> (-50.5, 13)
  line L9 (-50.5, 13) -> (-24.5, 13)
  line L10 (-24.5, 13) -> (-24.5, 10)
  line L11 (-24.5, 10) -> (-21.5, 10)
  line L12 (-21.5, 10) -> (-21.5, 13)
  line L13 (-21.5, 13) -> (4.5, 13)
  line L14 (4.5, 13) -> (4.5, 10)
  line L15 (4.5, 10) -> (7.5, 10)
  line L16 (7.5, 10) -> (7.5, 13)
  line L17 (7.5, 13) -> (33.5, 13)
  line L18 (33.5, 13) -> (33.5, 10)
  line L19 (33.5, 10) -> (36.5, 10)
  line L20 (36.5, 10) -> (36.5, 13)
  line L21 (36.5, 13) -> (55, 13)
  line L22 (55, 13) -> (55, 18)
  line L23 (55, 18) -> (58, 18)
  line L24 (58, 18) -> (58, 21)
  line L25 (58, 21) -> (55, 21)
  line L26 (55, 21) -> (55, 36.4645)
  line L27 (-81, 30.2322) -> (-81, 27.2322)
  line L28 (-81, 30.2322) -> (-84, 30.2322)
  line L29 (-81, 27.2322) -> (-84, 27.2322)
  line L30 (-84, 30.2322) -> (-84, 44.4645)
  line L31 (-84, 27.2322) -> (-84, 13)
  line L32 (-84, 30.2322) -> (-81, 30.2322)
  line L33 (-81, 30.2322) -> (-81, 27.2322)
  line L34 (-81, 27.2322) -> (-84, 27.2322)
  line L35 (-84, 44.4645) -> (-84, 30.2322)
  line L36 (-78, 16.2941) -> (-60, 16.2941)
  line L37 (-60, 16.2941) -> (-60, 15)
  line L38 (-60, 15) -> (-78, 15)
  line L39 (-78, 15) -> (-78, 16.2941)
  constraint vertical L27
  constraint perpendicular L27 L29
  constraint coincident L4.end L30.end
  constraint vertical L30
  constraint coincident L5.start L31.end
  constraint perpendicular L5 L31
extrude "Extrude48" add sketch "Sketch20" along normal blind 3 separate body makes body 48
ref_plane "WorkPlane20" through (-56.5, 9.5355, 48) normal (0, -0.707107, 0.707107) x (0, -0.707107, -0.707107)
sketch "Sketch21" plane through (0, -19.2322, 19.2322) normal (0, -0.707107, 0.707107) x (0, -0.707107, -0.707107)
  line L0 (-42.1838, -58) -> (-42.1838, -55)
  line L1 (-39.1838, -58) -> (-39.1838, -55)
  line L2 (-42.1838, -58) -> (-39.1838, -58)
  line L3 (-39.1838, -55) -> (-35.6838, -55)
  line L4 (-42.1838, -55) -> (-45.6838, -55)
  line L5 (-45.6838, -55) -> (-45.6838, 84)
  line L6 (-35.6838, -55) -> (-35.6838, 84)
  line L7 (-39.1838, 81) -> (-42.1838, 81)
  line L8 (-42.1838, 81) -> (-42.1838, 84)
  line L9 (-39.1838, 81) -> (-39.1838, 84)
  line L10 (-35.6838, 84) -> (-39.1838, 84)
  line L11 (-42.1838, 84) -> (-45.6838, 84)
  dimension "d365" = 3.5
  dimension "d366" = 3.5
  dimension "d367" = 139
  dimension "d368" = 139
  dimension "d405" = 3
  constraint coincident L1.end L3.start
  constraint perpendicular L1 L3
  constraint coincident L0.end L4.start
  constraint perpendicular L0 L4
  constraint perpendicular L4 L5
  constraint perpendicular L3 L6
  constraint horizontal L7
  constraint perpendicular L7 L8
  constraint perpendicular L9 L10
  constraint collinear L10 L11
  measures "d365" distance of L1.end L3.end
  measures "d366" distance of L0.end L4.end
  measures "d367" distance of L4.end L5.end
  measures "d368" distance of L3.end L6.end
  measures "d405" distance of L7.start L7.end
extrude "Extrude49" add sketch "Sketch21" along normal blind 3 separate body makes body 49
ref_plane "WorkPlane21" through (-56.5, 44.4645, 48) normal (0, 0.707107, 0.707107) x (0, -0.707107, 0.707107)
sketch "Sketch22" plane through (0, 46.2322, 46.2322) normal (0, 0.707107, 0.707107) x (0, -0.707107, 0.707107)
  line L0 (4, -58) -> (4, -55)
  line L1 (1, -58) -> (1, -55)
  line L2 (1, -58) -> (4, -58)
  line L3 (4, -55) -> (7.5, -55)
  line L4 (7.5, -55) -> (7.5, 84)
  line L5 (1, -55) -> (-2.5, -55)
  line L6 (-2.5, -55) -> (-2.5, 84)
  line L7 (4, 81) -> (1, 81)
  line L8 (1, 81) -> (1, 84)
  line L9 (4, 81) -> (4, 84)
  line L10 (7.5, 84) -> (4, 84)
  line L11 (1, 84) -> (-2.5, 84)
  dimension "d372" = 3.5
  dimension "d373" = 139
  dimension "d374" = 3.5
  dimension "d375" = 139
  constraint coincident L0.end L3.start
  constraint perpendicular L0 L3
  constraint perpendicular L3 L4
  constraint coincident L1.end L5.start
  constraint perpendicular L1 L5
  constraint perpendicular L5 L6
  constraint horizontal L7
  constraint coincident L8.end L10
  constraint perpendicular L8 L10
  constraint perpendicular L9 L10
  constraint collinear L10 L11
  measures "d372" distance of L0.end L3.end
  measures "d373" distance of L3.end L4.end
  measures "d374" distance of L1.end L5.end
  measures "d375" distance of L5.end L6.end
extrude "Extrude50" add sketch "Sketch22" along normal blind 3 separate body makes body 50
ref_plane "WorkPlane22" through (-56.5, 36.9897, 52.2301) normal (0, 0.173648, 0.984808) x (0, -0.984808, 0.173648)
sketch "Sketch23" plane through (0, 10.0473, 56.9808) normal (0, 0.173648, 0.984808) x (0, -0.984808, 0.173648)
  line L0 (-25.8581, -58) -> (-25.8581, -55)
  line L1 (-28.8581, -58) -> (-25.8581, -58)
  line L2 (-28.8581, -58) -> (-28.8581, -55)
  line L3 (-28.8581, -55) -> (-31.3581, -55)
  line L4 (-25.8581, -55) -> (-23.3581, -55)
  line L5 (-31.3581, -55) -> (-31.3581, 84)
  line L6 (-23.3581, -55) -> (-23.3581, 84)
  line L7 (-25.8581, 81) -> (-28.8581, 81)
  line L8 (-28.8581, 81) -> (-28.8581, 84)
  line L9 (-25.8581, 81) -> (-25.8581, 84)
  line L10 (-31.3581, 84) -> (-28.8581, 84)
  line L11 (-25.8581, 84) -> (-23.3581, 84)
  dimension "d379" = 2.5
  dimension "d380" = 2.5
  dimension "d381" = 139
  dimension "d382" = 139
  dimension "d407" = 3
  constraint coincident L2.end L3.start
  constraint perpendicular L2 L3
  constraint coincident L0.end L4.start
  constraint perpendicular L0 L4
  constraint perpendicular L3 L5
  constraint perpendicular L4 L6
  constraint horizontal L7
  constraint perpendicular L8 L10
  constraint coincident L9.end L10
  constraint perpendicular L9 L10
  constraint collinear L10 L11
  measures "d379" distance of L2.end L3.end
  measures "d380" distance of L0.end L4.end
  measures "d381" distance of L3.end L5.end
  measures "d382" distance of L4.end L6.end
  measures "d407" distance of L7.start L7.end
extrude "Extrude51" add sketch "Sketch23" along normal blind 3 separate body makes body 51
ref_plane "WorkPlane23" through (-56.5, 17.0103, 52.2301) normal (0, -0.173648, 0.984808) x (0, -0.984808, -0.173648)
sketch "Sketch24" plane through (0, -8.419, 47.7463) normal (0, -0.173648, 0.984808) x (0, -0.984808, -0.173648)
  line L0 (-27.3215, -58) -> (-27.3215, -55)
  line L1 (-27.3215, -58) -> (-24.3215, -58)
  line L2 (-24.3215, -58) -> (-24.3215, -55)
  line L3 (-24.3215, -55) -> (-21.8215, -55)
  line L4 (-27.3215, -55) -> (-29.8215, -55)
  line L5 (-21.8215, -55) -> (-21.8215, 84)
  line L6 (-29.8215, -55) -> (-29.8215, 84)
  line L7 (-24.3215, 81) -> (-27.3215, 81)
  line L8 (-27.3215, 81) -> (-27.3215, 84)
  line L9 (-24.3215, 81) -> (-24.3215, 84)
  line L10 (-29.8215, 84) -> (-27.3215, 84)
  line L11 (-24.3215, 84) -> (-21.8215, 84)
  dimension "d386" = 2.5
  dimension "d387" = 2.5
  dimension "d388" = 139
  dimension "d389" = 139
  dimension "d406" = 3
  constraint coincident L2.end L3.start
  constraint perpendicular L2 L3
  constraint coincident L0.end L4.start
  constraint perpendicular L0 L4
  constraint perpendicular L3 L5
  constraint perpendicular L4 L6
  constraint horizontal L7
  constraint perpendicular L8 L10
  constraint coincident L9.end L10
  constraint perpendicular L9 L10
  constraint collinear L10 L11
  measures "d386" distance of L2.end L3.end
  measures "d387" distance of L0.end L4.end
  measures "d388" distance of L3.end L5.end
  measures "d389" distance of L4.end L6.end
  measures "d406" distance of L7.start L7.end
extrude "Extrude52" add sketch "Sketch24" along normal blind 3 separate body makes body 52
ref_plane "WorkPlane24" through (-56.5, 27, 52.9247) normal (0, 0, 1) x (0, -1, 0)